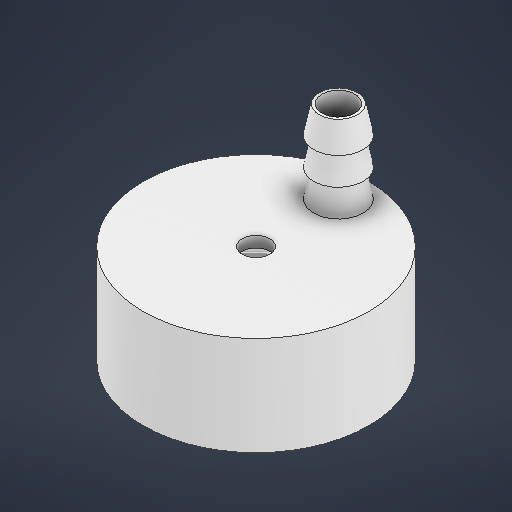
# Autodesk Inventor part: Cap
Saved by Autodesk Inventor 2027 (Build 310192060, 192F)
## iProperties
Created: 2026-08-20
Part Number: Cap
Material: PPS Plastic
Document SubType Name: Modeling
Designer: trtrn
Density: 1.637 g/cm^3
Appearance: Smooth - White
Author: trtrn
Autodesk Inventor part; units mm, degrees
ref_plane "YZ Plane" through (0, 0, 0) normal (1, 0, 0) x (0, 1, 0)
ref_plane "XZ Plane" through (0, 0, 0) normal (0, 1, 0) x (-1, 0, 0)
sketch "Sketch1" plane through (0, 0, 0) normal (0, 1, 0) x (-1, 0, 0)
  circle A0 centre (0, 0) radius 19.5
  circle A1 centre (0, 0) radius 20.5
  dimension "d0" = 39
  dimension "d1" = 41
  constraints: 2 centre point, 2 coincident
  measures "d0" diameter of A0
  measures "d1" diameter of A1
extrude "Extrusion1" add sketch "Sketch1" along normal blind 16
thread "Thread1" size "M39x2" class "6H" standard "ANSI Metric M Profile" length 16
sketch "Sketch2" plane through (0, 16, 0) normal (0, 1, 0) x (1, 0, 0)
  circle A0 centre (0, 0) radius 20.5
  circle A1 centre (0, 0) radius 20.5 projected
  constraints: 1 centre point, 1 coincident, 1 concentric
extrude "Extrusion2" add sketch "Sketch2" along normal blind 2
sketch "Sketch3" plane through (0, 18, 0) normal (0, 1, 0) x (1, 0, 0)
  circle A0 centre (0, 0) radius 2.5
  dimension "d8" = 5
  constraints: 1 centre point, 1 coincident
  measures "d8" diameter of A0
extrude "Extrusion3" cut sketch "Sketch3" against normal blind 2
sketch "Sketch4" plane through (0, 18, 0) normal (0, 1, 0) x (1, 0, 0)
  circle A0 centre (0, 15) radius 4.5
  point P0 (0, 0)
  dimension "d13" = 9
  dimension "d14" = 15
  constraints: 1 centre point, 1 vertical alignment
  measures "d13" diameter of A0
  measures "d14" distance of point (0, 0) A0.centre
ref_plane "Work Plane1" through (0, 23, 0) normal (0, 1, 0) x (1, 0, 0)
sketch "Sketch5" plane through (0, 23, 0) normal (0, 1, 0) x (1, 0, 0)
  circle A0 centre (0, 15) radius 3.5
  point P0 (0, 0)
  dimension "d16" = 7
  constraints: 1 centre point, 1 coincident
  measures "d16" diameter of A0
loft "Loft1" add profiles "Sketch4", "Sketch5"
pattern_linear "Rectangular Pattern2" count 3 spacing 5 along (0, 1, 0) of "Loft1"
sketch "Sketch9" plane through (0, 33, -15) normal (0, 1, 0) x (1, 0, 0)
  circle A0 centre (0, 0) radius 3
  circle A1 centre (0, 0) radius 3.5 projected
  point P0 (0, -15)
  dimension "d33" = 6
  constraints: 1 centre point, 1 concentric
  measures "d33" diameter of A0
extrude "Extrusion5" cut sketch "Sketch9" against normal through all contours A0
body "Solid1"
